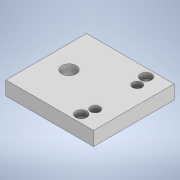
# Autodesk Inventor part: Linear Rail End Cap
Saved by Autodesk Inventor 2022 (Build 260153000, 153)
## iProperties
Created: 2021-11-30
Part Number: Linear Rail End Cap
Material: Generic
Document SubType Name: Modeling
Designer: efred
Density: 1 g/cm^3
Appearance: Default
Author: efred
Autodesk Inventor part; units mm, degrees
ref_plane "YZ Plane" through (0, 0, 0) normal (1, 0, 0) x (0, 1, 0)
ref_plane "XZ Plane" through (0, 0, 0) normal (0, 1, 0) x (-1, 0, 0)
ref_plane "XY Plane" through (0, 0, 0) normal (0, 0, 1) x (1, 0, 0)
sketch "Sketch1" plane through (0, 0, 0) normal (0, 1, 0) x (-1, 0, 0)
  line L0 (-25, 23) -> (25, 23)
  line L1 (25, 23) -> (25, -23)
  line L2 (25, -23) -> (-25, -23)
  line L3 (-25, -23) -> (-25, 23)
  line L4 (-25, 23) -> (25, -23) construction
  line L5 (25, 23) -> (-25, -23) construction
  circle A0 centre (12, 0) radius 4.15
  circle A1 centre (-15, -12) radius 2.65
  line L6 (25, 0) -> (-25, 0) construction
  circle A2 centre (-15, 12) radius 2.65
  point P0 (0, 0)
  dimension "d0" = 46
  dimension "d1" = 50
  dimension "d2" = 23
  dimension "d3" = 13
  dimension "d4" = 8.3
  dimension "d5" = 11
  dimension "d6" = 10
  dimension "d7" = 5.3
  constraints: 14 end point, 4 midpoint, 3 centre point, 2 parallel, 1 horizontal, 1 perpendicular, 1 symmetric about line, 1 other
  measures "d0" distance of L0.end L1.end
  measures "d1" distance of L1.end L2.end
  measures "d2" distance from line of L2 A0.centre
  measures "d3" distance from line of L1 A0.centre
  measures "d4" diameter of A0
  measures "d5" distance from line of L2 A1.centre
  measures "d6" distance from line of L3 A1.centre
  measures "d7" diameter of A1
extrude "Extrusion1" add sketch "Sketch1" along normal blind 8
sketch "Sketch2" plane through (0, 0, 0) normal (0, -1, 0) x (1, 0, 0)
  line L0 (25, -23) -> (-25, -23) projected
  line L1 (25, 23) -> (25, -23) projected
  line L2 (-25, 23) -> (25, 23) projected
  line L3 (-25, -23) -> (-25, 23) projected
  circle A0 centre (15, 12) radius 2.65 construction
  circle A1 centre (15, -12) radius 2.65 construction
  circle A2 centre (-12, 0) radius 4.15 projected
  circle A3 centre (15, -12) radius 2.65 construction
  circle A4 centre (15, -12) radius 5
  circle A5 centre (15, 12) radius 5
  point P0 (0, 0)
  dimension "d10" = 10
  dimension "d11" = 10
  constraints: 2 centre point, 2 coincident
  measures "d10" diameter of A4
  measures "d11" diameter of A5
extrude "Extrusion2" cut sketch "Sketch2" against normal blind 5 contours A4 | A5
sketch "Sketch3" plane through (0, 8, 0) normal (0, 1, 0) x (1, 0, 0)
  circle A0 centre (13.5, 18.5) radius 3.15
  line L0 (25, -23) -> (25, 23) projected
  line L1 (25, 0) -> (-25, 0) construction
  line L2 (-25, 23) -> (-25, -23) projected
  line L3 (25, 23) -> (-25, 23) projected
  circle A1 centre (13.5, -18.5) radius 3.15
  point P0 (0, 0)
  dimension "d14" = 4.5
  dimension "d15" = 11.5
  dimension "d16" = 6.3
  constraints: 2 centre point, 2 end point, 2 midpoint, 1 symmetric about line, 1 other
  measures "d14" distance from line of L3 A0.centre
  measures "d15" distance from line of L0 A0.centre
  measures "d16" diameter of A0
extrude "Extrusion3" cut sketch "Sketch3" against normal blind 3
sketch "Sketch5" plane through (0, 0, 0) normal (0, -1, 0) x (1, 0, 0)
  circle A0 centre (-12, 0) radius 4.15 projected
  point P0 (0, 0)
extrude "Extrusion5" add sketch "Sketch5" against normal blind 1
equation "\"d11\" = d10"
body "Solid1"
